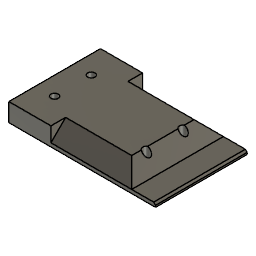
right cover merger (Autodesk Fusion 360 design; units mm, degrees)
Autodesk Fusion 360 part; units mm, degrees
note: some values were not read from the file. Chosen so that the rebuilt part matches the saved one: which bodies a step acts on.
sketch "Szkic1" plane through (0, 0, 0) normal (0, 0, 1) x (1, 0, 0)
  line L0 (-35, 265) -> (-35, 0)
  line L1 (-35, 0) -> (45, 0)
  circle A0 centre (-25, 60) radius 1.75
  circle A1 centre (-25, -60) radius 1.75
  line L2 (45, 0) -> (-35, 0)
  line L3 (-35, 0) -> (-35, -230)
  circle A2 centre (-25, -10) radius 3.5
  circle A3 centre (25, -10) radius 3.5
  circle A4 centre (25, 10) radius 3.5
  circle A5 centre (-25, 10) radius 3.5
  line L4 (45, 25) -> (45, -25)
  line L5 (-35, 0) -> (-12, 0)
  line L6 (-12, 0) -> (-12, -25)
  line L7 (-12, -25) -> (-35, -25)
  line L8 (-35, -25) -> (-35, 0)
  line L9 (-35, 0) -> (-12, 0)
  line L10 (-12, 0) -> (-12, 25)
  line L11 (-12, 25) -> (-35, 25)
  line L12 (-35, 25) -> (-35, 0)
  line L13 (-12, -25) -> (45, -25)
  line L14 (-12, 25) -> (45, 25)
  circle A6 centre (-25, 10) radius 2
  circle A7 centre (-25, -10) radius 2
  circle A8 centre (25, -10) radius 2
  circle A9 centre (25, 10) radius 2
  dimension "d1" = 7
  dimension "d2" = 7
  dimension "d3" = 7
  dimension "d4" = 7
  dimension "d5" = 4
  dimension "d6" = 4
  dimension "d7" = 4
  dimension "d8" = 4
  constraint vertical L4
  constraint perpendicular L5 L6
  constraint parallel L5 L7
  constraint parallel L6 L8
  constraint perpendicular L0 L5
  constraint perpendicular L9 L10
  constraint parallel L9 L11
  constraint parallel L10 L12
  constraint perpendicular L4 L13
  constraint perpendicular L4 L14
  constraint concentric A5 A6
  constraint concentric A2 A7
  constraint concentric A3 A8
  constraint concentric A4 A9
  measures "d1" diameter of A2
  measures "d2" diameter of A3
  measures "d3" diameter of A4
  measures "d4" diameter of A5
  measures "d5" diameter of A6
  measures "d6" diameter of A7
  measures "d7" diameter of A8
  measures "d8" diameter of A9
extrude "Wyciągnięcie proste1" add sketch "Szkic1" along normal blind 10 contours L0 L1 L2 L5 L9 L10 L11 L12 | L1 L2 L3 L5 L6 L7 L8 L9 | L1 L2 L4 L10 L14 | L1 L2 L4 L6 L13 | A2 | A3 | A4 | A5 makes body 1
extrude "Wyciągnięcie proste2" cut sketch "Szkic1" along normal blind 12 contours L0 L1 L2 L5 L9 L10 L11 L12 | L1 L2 L3 L5 L6 L7 L8 L9 bodies 1 makes body 2 at (-21.5174, -9.6515, 6.6667) makes body 3 at (-0.3037, -3.1368, 0)
chamfer "Fazowanie1" distance 8 angle 45 1 edges at (16.5, -25, 10) on bodies 3
chamfer "Fazowanie2" distance 8 angle 45 1 edges at (16.5, 25, 10) on bodies 3
extrude "Wyciągnięcie proste3" add sketch "Szkic1" along normal blind 10 contours L0 L1 L2 L5 L9 L10 L11 L12 | L1 L2 L3 L5 L6 L7 L8 L9 bodies 1 2 3
chamfer "Fazowanie3" distance 8 angle 45 1 edges at (45, 0, 10) on bodies 1
delete_face "Usuń powierzchnię1" 1 faces at (42.3333, 5.6667, 4.6667) on bodies 1
extrude "Wyciągnięcie proste4" cut 1 faces at (45, 5.6667, 3.3333) along direction (-1, 0, 0) blind 13 on bodies 1 bodies 1
chamfer "Fazowanie4" distance 8 angle 45 1 edges at (32, 0, 10) on bodies 1
extrude "Wyciągnięcie proste5" add 1 faces at (32, 8.3333, 0.6667) along direction (1, 0, 0) blind 13 on bodies 1 bodies 1
chamfer "Fazowanie5" distance 1 angle 45 1 edges at (45, 0, 2) on bodies 1
